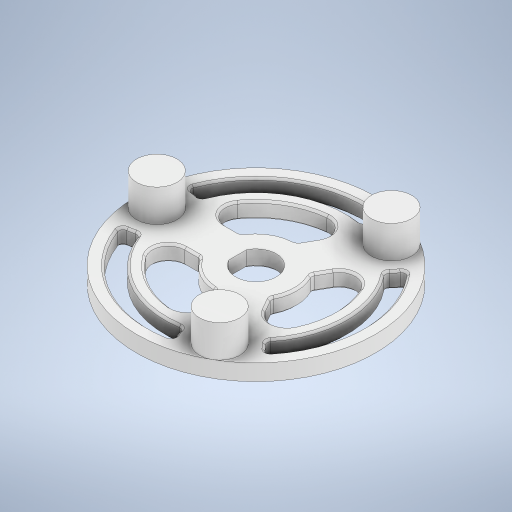
# Autodesk Inventor part: insert
Saved by Autodesk Inventor 2023 (Build 270158000, 158)
## iProperties
Created: 2022-12-06
Part Number: insert
Material: Acetal Resin, White
Document SubType Name: Modeling
Designer: Owner
Density: 1.425 g/cm^3
Appearance: Smooth - White
Mass: 2.2255 g
Surface Area: 17.3109 cm^2
Volume: 1.56175 cm^3
Author: Owner
Autodesk Inventor part; units mm, degrees
ref_plane "YZ Plane" through (0, 0, 0) normal (1, 0, 0) x (0, 1, 0)
ref_plane "XZ Plane" through (0, 0, 0) normal (0, 1, 0) x (-1, 0, 0)
ref_plane "XY Plane" through (0, 0, 0) normal (0, 0, 1) x (1, 0, 0)
sketch "Sketch1" plane through (0, 0, 0) normal (0, 1, 0) x (-1, 0, 0)
  line L0 (15.55, 0) -> (21.15, 0) construction
  line L1 (18.35, 0) -> (21.15, 0) construction
  arc A0 (2.25, 1.0897) -> (2.25, -1.0897) centre (0, 0) ccw construction
  circle A1 centre (0, 0) radius 2.25 construction
  line L2 (2.25, 0) -> (2.25, 1.0897) construction
  line L3 (2.25, 0) -> (2.25, -1.0897) construction
  line L4 (-15.5, 21.15) -> (15.5, 21.15) construction
  line L5 (21.15, 15.5) -> (21.15, -15.5) construction
  line L6 (15.5, -21.15) -> (-15.5, -21.15) construction
  line L7 (-21.15, -15.5) -> (-21.15, 15.5) construction
  line L8 (-21.15, 21.15) -> (21.15, -21.15) construction
  line L9 (21.15, 21.15) -> (-21.15, -21.15) construction
  line L10 (-15.5, 15.5) -> (15.5, 15.5) construction
  line L11 (15.5, 15.5) -> (15.5, -15.5) construction
  line L12 (15.5, -15.5) -> (-15.5, -15.5) construction
  line L13 (-15.5, -15.5) -> (-15.5, 15.5) construction
  line L14 (-15.5, 15.5) -> (15.5, -15.5) construction
  line L15 (15.5, 15.5) -> (-15.5, -15.5) construction
  circle A2 centre (15.5, 15.5) radius 1.625 construction
  circle A3 centre (15.5, -15.5) radius 1.625 construction
  circle A4 centre (-15.5, -15.5) radius 1.625 construction
  circle A5 centre (-15.5, 15.5) radius 1.625 construction
  line L16 (15.5, -15.5) -> (15.5, -21.15) construction
  line L17 (21.15, -15.5) -> (15.5, -21.15) construction
  line L18 (-15.5, -21.15) -> (-21.15, -15.5) construction
  line L19 (-21.15, 15.5) -> (-15.5, 21.15) construction
  line L20 (15.5, 21.15) -> (21.15, 15.5) construction
  line L21 (0, -15.5) -> (0, -21.15) construction
  line L22 (0, -15.5) -> (0, -18.325) construction
  line L23 (0, -18.325) -> (0, -21.15) construction
  circle A6 centre (0, 0) radius 19.7375 construction
  line L24 (-15.5, -21.15) -> (15.5, -21.15) construction
  line L25 (-13.9565, -13.9565) -> (-6.763, -21.15) construction
  line L26 (0, 0) -> (7.7782, -7.7782) construction
  line L27 (13.9565, 13.9565) -> (21.15, 6.763) construction
  line L28 (-1.1373, -19.7047) -> (0.308, -21.15) construction
  line L29 (19.7047, 1.1373) -> (21.15, -0.308) construction
  arc A7 (2.25, 1.0897) -> (2.25, -1.0897) centre (0, 0) ccw
  line L30 (2.25, 1.0897) -> (2.25, -1.0897)
  circle A8 centre (0, 0) radius 3.75
  line L31 (-19.7375, 0) -> (-17.7375, 0)
  line L32 (-19.7375, 0) -> (-14.7375, 0)
  line L33 (-17.7375, 0) -> (-6.7375, 0)
  circle A9 centre (-12.2375, 0) radius 5.5 construction
  circle A10 centre (-12.2375, 0) radius 2.5
  line L34 (-12.2375, 2.5) -> (-1.8548, 2.5) construction
  line L35 (-12.2375, -2.5) -> (-1.8548, -2.5) construction
  line L36 (3.9537, -11.848) -> (-1.2377, -2.8563) construction
  circle A11 centre (6.1187, -10.598) radius 2.5
  line L37 (8.2838, -9.348) -> (3.0924, -0.3563) construction
  circle A12 centre (6.1187, -10.598) radius 5.5 construction
  line L38 (8.2838, 9.348) -> (3.0924, 0.3563) construction
  circle A13 centre (6.1188, 10.598) radius 2.5
  line L39 (3.9537, 11.848) -> (-1.2377, 2.8563) construction
  circle A14 centre (6.1188, 10.598) radius 5.5 construction
  circle A15 centre (0, 0) radius 14.7375
  circle A16 centre (0, 0) radius 9.7375
  point P0 (-10.421, -10.421)
  point P1 (10.421, 10.421)
  point P2 (20.4274, 0.4146)
  point P3 (15.5, 12.2196)
  point P4 (15.5, 12.413)
  point P5 (-12.413, -15.5)
  point P6 (-12.2196, -15.5)
  point P7 (0, -20.842)
  point P8 (21.15, -0.308)
  point P9 (3.3687, -5.8348)
  point P10 (3.3688, 5.8348)
  dimension "d9" = 4.5
  dimension "d8" = 5
  dimension "d10" = 42.3
  dimension "d11" = 42.3
  dimension "d12" = 31
  dimension "d13" = 31
  dimension "d15" = 3.25
  dimension "d16" = 3.25
  dimension "d17" = 3.25
  dimension "d18" = 3.25
  dimension "d20" = 5
  dimension "d21" = 7.5
  dimension "d22" = 2
  dimension "d23" = 5
  dimension "d24" = 11
  dimension "d25" = 5
  dimension "d28" = 360
  dimension "d31" = 5
  constraints: 80 end point, 14 point on circle, 12 centre point, 11 coincident, 10 midpoint, 10 point on line, 7 perpendicular, 6 horizontal, 4 parallel, 4 symmetric about line, 3 collinear, 3 horizontal alignment, 2 tangent, 2 vertical, 1 concentric, 46 other
  measures "d8" diameter of A0
  measures "d10" distance of L8.end L9.end
  measures "d11" distance of L9.start L8.end
  measures "d12" distance of L11.end L12.end
  measures "d13" distance of L10.end L11.end
  measures "d15" diameter of A2
  measures "d16" diameter of A3
  measures "d17" diameter of A4
  measures "d18" diameter of A5
  measures "d20" distance from line of point (20.427, 0.415) L27
  measures "d21" diameter of A8
  measures "d22" distance of L31.start L31.end
  measures "d23" distance of L31.start L32.end
  measures "d24" distance of L31.end L33.end
  measures "d25" diameter of A10
extrude "Extrusion1" add sketch "Sketch1" along normal blind 2 contours A8 | A10 L33 | A15 A13 A16 A10 | L33 A10 | A10 A16 A11 A15 | A16 | A15 A11 A16 A13 | A13 | A11
sketch "Sketch2" plane through (0, 2, 0) normal (0, 1, 0) x (1, 0, 0)
  line L0 (15.55, 0) -> (21.15, 0) construction
  line L1 (18.35, 0) -> (21.15, 0) construction
  arc A0 (2.25, 1.0897) -> (2.25, -1.0897) centre (0, 0) ccw construction
  circle A1 centre (0, 0) radius 2.25 construction
  line L2 (2.25, 0) -> (2.25, 1.0897) construction
  line L3 (2.25, 0) -> (2.25, -1.0897) construction
  line L4 (-15.5, 21.15) -> (15.5, 21.15) construction
  line L5 (21.15, 15.5) -> (21.15, -15.5) construction
  line L6 (15.5, -21.15) -> (-15.5, -21.15) construction
  line L7 (-21.15, -15.5) -> (-21.15, 15.5) construction
  line L8 (-21.15, 21.15) -> (21.15, -21.15) construction
  line L9 (21.15, 21.15) -> (-21.15, -21.15) construction
  line L10 (-15.5, 15.5) -> (15.5, 15.5) construction
  line L11 (15.5, 15.5) -> (15.5, -15.5) construction
  line L12 (15.5, -15.5) -> (-15.5, -15.5) construction
  line L13 (-15.5, -15.5) -> (-15.5, 15.5) construction
  line L14 (-15.5, 15.5) -> (15.5, -15.5) construction
  line L15 (15.5, 15.5) -> (-15.5, -15.5) construction
  circle A2 centre (15.5, 15.5) radius 1.625 construction
  circle A3 centre (15.5, -15.5) radius 1.625 construction
  circle A4 centre (-15.5, -15.5) radius 1.625 construction
  circle A5 centre (-15.5, 15.5) radius 1.625 construction
  line L16 (15.5, -15.5) -> (15.5, -21.15) construction
  line L17 (21.15, -15.5) -> (15.5, -21.15) construction
  line L18 (-15.5, -21.15) -> (-21.15, -15.5) construction
  line L19 (-21.15, 15.5) -> (-15.5, 21.15) construction
  line L20 (15.5, 21.15) -> (21.15, 15.5) construction
  line L21 (0, -15.5) -> (0, -21.15) construction
  line L22 (0, -15.5) -> (0, -18.325) construction
  line L23 (0, -18.325) -> (0, -21.15) construction
  circle A6 centre (0, 0) radius 19.7375 construction
  line L24 (-15.5, -21.15) -> (15.5, -21.15) construction
  line L25 (-13.9565, -13.9565) -> (-6.763, -21.15) construction
  line L26 (0, 0) -> (7.7782, -7.7782) construction
  line L27 (13.9565, 13.9565) -> (21.15, 6.763) construction
  line L28 (-1.1373, -19.7047) -> (0.308, -21.15) construction
  line L29 (19.7047, 1.1373) -> (21.15, -0.308) construction
  arc A7 (2.25, 1.0897) -> (2.25, -1.0897) centre (0, 0) ccw
  line L30 (2.25, 1.0897) -> (2.25, -1.0897)
  circle A8 centre (0, 0) radius 3.75
  line L31 (-19.7375, 0) -> (-17.7375, 0)
  line L32 (-19.7375, 0) -> (-14.7375, 0)
  line L33 (-17.7375, 0) -> (-6.7375, 0)
  circle A9 centre (-12.2375, 0) radius 5.5 construction
  circle A10 centre (-12.2375, 0) radius 2.5
  line L34 (-12.2375, 2.5) -> (-1.8548, 2.5) construction
  line L35 (-12.2375, -2.5) -> (-1.8548, -2.5) construction
  line L36 (3.9537, -11.848) -> (-1.2377, -2.8563) construction
  circle A11 centre (6.1187, -10.598) radius 2.5
  line L37 (8.2838, -9.348) -> (3.0924, -0.3563) construction
  circle A12 centre (6.1187, -10.598) radius 5.5 construction
  line L38 (8.2838, 9.348) -> (3.0924, 0.3563) construction
  circle A13 centre (6.1188, 10.598) radius 2.5
  line L39 (3.9537, 11.848) -> (-1.2377, 2.8563) construction
  circle A14 centre (6.1188, 10.598) radius 5.5 construction
  circle A15 centre (0, 0) radius 14.7375
  circle A16 centre (0, 0) radius 9.7375
  point P0 (-10.421, -10.421)
  point P1 (20.4274, 0.4146)
  point P2 (10.421, 10.421)
  point P3 (15.5, 12.2196)
  point P4 (15.5, 12.413)
  point P5 (-12.413, -15.5)
  point P6 (-12.2196, -15.5)
  point P7 (0, -20.842)
  point P8 (21.15, -0.308)
  point P9 (3.3687, -5.8348)
  point P10 (3.3688, 5.8348)
  dimension "d37" = 4.5
  dimension "d36" = 5
  dimension "d38" = 42.3
  dimension "d39" = 42.3
  dimension "d40" = 31
  dimension "d41" = 31
  dimension "d42" = 3.25
  dimension "d43" = 3.25
  dimension "d44" = 3.25
  dimension "d45" = 3.25
  dimension "d46" = 5
  dimension "d47" = 7.5
  dimension "d48" = 2
  dimension "d49" = 5
  dimension "d50" = 11
  dimension "d51" = 5
  dimension "d52" = 360
  dimension "d53" = 5
  constraints: 80 end point, 14 point on circle, 12 centre point, 11 coincident, 10 midpoint, 10 point on line, 7 perpendicular, 6 horizontal, 4 parallel, 4 symmetric about line, 3 collinear, 3 horizontal alignment, 2 tangent, 2 vertical, 1 concentric, 46 other
  measures "d36" diameter of A0
  measures "d38" distance of L8.end L9.end
  measures "d39" distance of L9.start L8.end
  measures "d40" distance of L11.end L12.end
  measures "d41" distance of L10.end L11.end
  measures "d42" diameter of A2
  measures "d43" diameter of A3
  measures "d44" diameter of A4
  measures "d45" diameter of A5
  measures "d46" distance from line of point (20.427, 0.415) L27
  measures "d47" diameter of A8
  measures "d48" distance of L31.start L31.end
  measures "d49" distance of L31.start L32.end
  measures "d50" distance of L31.end L33.end
  measures "d51" diameter of A10
extrude "Extrusion2" add sketch "Sketch2" along normal blind 4 contours A10 L33 | L33 A10 | A13 | A11
sketch "Sketch4" plane through (6.1187, 2, 10.598) normal (0, 1, 0) x (1, 0, 0)
  circle A0 centre (-6.1187, 10.598) radius 14.7375 projected
  arc A1 (-14.0401, 4.9348) -> (-7.0625, 0.9063) centre (-6.1187, 10.598) ccw
  circle A2 centre (-18.3562, 10.598) radius 2.5 projected
  arc A3 (-20.8562, 10.598) -> (-15.8562, 10.598) centre (-18.3562, 10.598) ccw
  arc A4 (-1.25, 2.1651) -> (1.25, -2.1651) centre (0, 0) ccw
  arc A5 (-20.8562, 10.598) -> (1.25, -2.1651) centre (-6.1187, 10.598) ccw
  arc A6 (-3.8978, -0.8985) -> (-3.5964, -1.7509) centre (0, 0) ccw
  arc A7 (-18.507, 5.933) -> (-3.9646, -2.4631) centre (-6.1187, 10.598) ccw
  arc A8 (-16.5739, 6.4784) -> (-4.4589, -0.5162) centre (-6.1187, 10.598) ccw
  arc A9 (-18.0743, 6.6079) -> (-17.1854, 6.7732) centre (-18.3562, 10.598) ccw
  line L0 (-12.4131, 8.098) -> (-10.7285, 8.098)
  arc A10 (-8.3687, 9.5083) -> (-8.3687, 11.6877) centre (-6.1187, 10.598) ccw projected
  arc A11 (-12.4131, 8.098) -> (-14.0401, 4.9348) centre (-12.4131, 6.098) ccw
  arc A12 (-16.5739, 6.4784) -> (-17.1854, 6.7732) centre (-17.0391, 6.2951) ccw
  arc A13 (-18.0743, 6.6079) -> (-18.507, 5.933) centre (-18.0391, 6.1092) ccw
  arc A14 (-3.9646, -2.4631) -> (-3.5964, -1.7509) centre (-4.046, -1.9697) ccw
  arc A15 (-3.8978, -0.8985) -> (-4.4589, -0.5162) centre (-4.385, -1.0108) ccw
  arc A16 (-10.3095, 7.8707) -> (-10.7285, 8.098) centre (-10.7285, 7.598) ccw
  line L1 (-6.1187, 10.598) -> (-9.6187, 4.5358)
  line L2 (-6.1187, 10.598) -> (0.8813, 10.598) construction
  arc A17 (-14.0401, 4.9348) -> (-7.0625, 0.9063) centre (-6.1187, 10.598) ccw
  line L3 (-5.1366, 3.8969) -> (-5.9789, 5.3558)
  arc A18 (-7.0625, 0.9063) -> (-5.1366, 3.8969) centre (-6.8687, 2.8969) ccw
  arc A19 (-5.9789, 5.3558) -> (-6.3853, 5.6051) centre (-6.4119, 5.1058) ccw
  arc A20 (-10.3095, 7.8707) -> (-6.3853, 5.6051) centre (-6.1187, 10.598) ccw
  arc A21 (-10.3095, 7.8707) -> (-6.3853, 5.6051) centre (-6.1187, 10.598) ccw
  line L4 (-0.8065, 14.7991) -> (-1.6488, 13.3402)
  arc A22 (-1.6488, 13.3402) -> (-1.6615, 12.8636) centre (-1.2158, 13.0902) ccw
  line L5 (-6.1187, 10.598) -> (-9.6187, 16.6602) construction
  arc A23 (-1.6615, 8.3324) -> (-1.6615, 12.8636) centre (-6.1187, 10.598) ccw
  arc A24 (-1.6615, 8.3324) -> (-1.6615, 12.8636) centre (-6.1187, 10.598) ccw
  line L6 (-6.1187, 10.598) -> (0.8813, 10.598)
  arc A25 (2.7464, 6.5695) -> (2.7464, 14.6265) centre (-6.1187, 10.598) ccw
  arc A26 (2.7464, 6.5695) -> (2.7464, 14.6265) centre (-6.1187, 10.598) ccw
  arc A27 (1.25, -2.1651) -> (1.25, 23.361) centre (-6.1187, 10.598) ccw
  arc A28 (4.1154, 2.2019) -> (4.1154, 18.994) centre (-6.1187, 10.598) ccw
  arc A29 (2.6765, 3.6034) -> (2.6765, 17.5926) centre (-6.1187, 10.598) ccw
  line L7 (-0.8065, 6.3969) -> (-1.6488, 7.8558)
  arc A30 (1.25, -2.1651) -> (-1.25, 2.1651) centre (0, 0) ccw
  arc A31 (-1.6615, 8.3324) -> (-1.6488, 7.8558) centre (-1.2158, 8.1058) ccw
  arc A32 (3.3145, 2.2392) -> (2.727, 2.9264) centre (0, 0) ccw
  arc A33 (-0.8065, 6.3969) -> (2.7464, 6.5695) centre (0.9255, 7.3969) ccw
  arc A34 (2.6765, 3.6034) -> (2.727, 2.9264) centre (3.0679, 3.2922) ccw
  arc A35 (3.3145, 2.2392) -> (4.1154, 2.2019) centre (3.7288, 2.5191) ccw
  arc A36 (2.727, 18.2696) -> (3.3145, 18.9568) centre (0, 21.196) ccw
  arc A37 (2.727, 18.2696) -> (2.6765, 17.5926) centre (3.0679, 17.9038) ccw
  arc A38 (4.1154, 18.994) -> (3.3145, 18.9568) centre (3.7288, 18.6769) ccw
  arc A39 (-1.25, 19.0309) -> (1.25, 23.361) centre (0, 21.196) ccw
  arc A40 (2.7464, 14.6265) -> (-0.8065, 14.7991) centre (0.9255, 13.7991) ccw
  line L8 (-12.4131, 13.098) -> (-10.7285, 13.098)
  arc A41 (-10.7285, 13.098) -> (-10.3095, 13.3253) centre (-10.7285, 13.598) ccw
  line L9 (-6.1187, 10.598) -> (-9.6187, 4.5358) construction
  arc A42 (-6.3853, 15.5909) -> (-10.3095, 13.3253) centre (-6.1187, 10.598) ccw
  arc A43 (-6.3853, 15.5909) -> (-10.3095, 13.3253) centre (-6.1187, 10.598) ccw
  line L10 (-6.1187, 10.598) -> (-9.6187, 16.6602)
  arc A44 (-7.0625, 20.2896) -> (-14.0401, 16.2612) centre (-6.1187, 10.598) ccw
  arc A45 (-7.0625, 20.2896) -> (-14.0401, 16.2612) centre (-6.1187, 10.598) ccw
  arc A46 (1.25, 23.361) -> (-20.8562, 10.598) centre (-6.1187, 10.598) ccw
  arc A47 (-3.9646, 23.659) -> (-18.507, 15.263) centre (-6.1187, 10.598) ccw
  arc A48 (-4.4589, 21.7122) -> (-16.5739, 14.7176) centre (-6.1187, 10.598) ccw
  line L11 (-5.1366, 17.2991) -> (-5.9789, 15.8402)
  arc A49 (1.25, 23.361) -> (-1.25, 19.0309) centre (0, 21.196) ccw
  arc A50 (-6.3853, 15.5909) -> (-5.9789, 15.8402) centre (-6.4119, 16.0902) ccw
  arc A51 (-3.5964, 22.9468) -> (-3.8978, 22.0944) centre (0, 21.196) ccw
  arc A52 (-5.1366, 17.2991) -> (-7.0625, 20.2896) centre (-6.8687, 18.2991) ccw
  arc A53 (-4.4589, 21.7122) -> (-3.8978, 22.0944) centre (-4.385, 22.2067) ccw
  arc A54 (-3.5964, 22.9468) -> (-3.9646, 23.659) centre (-4.046, 23.1657) ccw
  arc A55 (-17.1854, 14.4228) -> (-18.0743, 14.588) centre (-18.3562, 10.598) ccw
  arc A56 (-17.1854, 14.4228) -> (-16.5739, 14.7176) centre (-17.0391, 14.9009) ccw
  arc A57 (-18.507, 15.263) -> (-18.0743, 14.588) centre (-18.0391, 15.0868) ccw
  arc A58 (-15.8562, 10.598) -> (-20.8562, 10.598) centre (-18.3562, 10.598) ccw
  arc A59 (-14.0401, 16.2612) -> (-12.4131, 13.098) centre (-12.4131, 15.098) ccw
  point P0 (-10.4489, 8.098)
  point P1 (-1.7886, 8.098)
  point P2 (-6.1187, 15.598)
  dimension "d60" = 2
  dimension "d62" = 0.5
  dimension "d63" = 4
  dimension "d64" = 13.2375
  dimension "d65" = 11.2375
  dimension "d67" = 0.5
  dimension "d68" = 7
  dimension "d69" = 120
  dimension "d70" = 5
  dimension "d71" = 8.4329
  dimension "d72" = 2.5
  dimension "d75" = 360
  constraints: 119 point on circle, 57 centre point, 24 end point, 17 tangent, 6 symmetric about line, 5 equal radius, 4 coincident, 3 point on line, 1 equal length, 1 horizontal, 1 horizontal alignment, 182 other
  measures "d60" radius of A11
  measures "d62" radius of A12
  measures "d63" radius of A6
  measures "d64" radius of A7
  measures "d65" radius of A8
  measures "d67" radius of A16
  measures "d68" distance of L1.start L1.end
  measures "d69" angle of L1 L2
  measures "d70" radius of A21
  measures "d71" distance from line of A4.start L2
  measures "d72" distance from line of point (-10.449, 8.098) L3
extrude "Extrusion3" cut sketch "Sketch4" against normal blind 3.75 contours A11 L0 A16 A20 A19 L3 A18 A1 | A6 A14 A7 A13 A9 A12 A8 A15 | A40 A25 A33 L7 A31 A23 A22 L4 | A35 A32 A34 A29 A37 A36 A38 A28 | A59 A44 A52 L11 A50 A42 A41 L8 | A54 A51 A53 A48 A56 A55 A57 A47
chamfer "Chamfer1" distance 0.25 angle 45 98 edges at (-6.6187, 2, -11.464) (2.5169, 2, -12.7973) (2.3475, 2, -11.9312) (2.0152, 2, -11.1955) (-5.6187, 2, -9.732) (-10.7032, 2, -3.8525) (-11.5065, 2, -3.9326) (-12.3413, 2, -4.219) (-4.8687, 2, -8.4329) (0.9316, 2, -8.7839) (0.561, 2, -5.9716) (-0.0317, 2, -5.066) (-2.5, 2, -4.3301) (-4.3714, 2, -2.5605) (-5.4521, 2, -2.5) (-8.0729, 2, -3.5852) (-8.0729, 2, 3.5852) (-5.4521, 2, 2.5) (-4.3714, 2, 2.5605) (-2.5, 2, 4.3301) (-0.0317, 2, 5.066) (0.561, 2, 5.9716) (0.9316, 2, 8.7839) (-4.8687, 2, 8.4329) (-11.5065, 2, 3.9326) (-10.7032, 2, 3.8525) (-5.6188, 2, 9.732) (2.0152, 2, 11.1955) (2.3475, 2, 11.9312) (2.5169, 2, 12.7973) (-6.6188, 2, 11.464) (-12.3413, 2, 4.219) (-11.5065, 0, 3.9326) (-12.3413, 0, 4.219) (-6.6188, 0, 11.464) (2.5169, 0, 12.7973) (2.3475, 0, 11.9312) (2.0152, 0, 11.1955) (-5.6187, 0, 9.732) (-10.7032, 0, 3.8525) (-8.0729, 0, 3.5852) (-4.8687, 0, 8.4329) (0.9316, 0, 8.7839) (0.561, 0, 5.9716) (-0.0317, 0, 5.066) (-2.5, 0, 4.3301) (-4.3714, 0, 2.5605) (-5.4521, 0, 2.5) (-4.8687, 0, -8.4329) (-8.0729, 0, -3.5852) (-5.4521, 0, -2.5) (-4.3714, 0, -2.5605) (-2.5, 0, -4.3301) (-0.0317, 0, -5.066) (0.561, 0, -5.9716) (0.9316, 0, -8.7839) (4.8911, 0, -3.4716) (4.4031, 0, -2.5055) (5, 0, 0) (4.4031, 0, 2.5055) (4.8911, 0, 3.4716) (7.1413, 0, 5.1987) (9.7375, 0, 0) (7.1413, 0, -5.1987) (4.8911, 2, -3.4716) (7.1413, 2, -5.1987) (9.7375, 2, 0) (7.1413, 2, 5.1987) (4.8911, 2, 3.4716) (4.4031, 2, 2.5055) (5, 2, 0) (4.4031, 2, -2.5055) (11.2375, 2, 0) (8.688, 2, -7.343) (9.159, 2, -7.9986) (9.8244, 2, -8.5784) (13.2375, 2, 0) (9.8244, 2, 8.5784) (9.159, 2, 7.9986) (8.688, 2, 7.343) (9.159, 0, -7.9986) (8.688, 0, -7.343) (11.2375, 0, 0) (8.688, 0, 7.343) (9.159, 0, 7.9986) (9.8244, 0, 8.5784) (13.2375, 0, 0) (9.8244, 0, -8.5784) (-6.6187, 0, -11.464) (-12.3413, 0, -4.219) (-11.5065, 0, -3.9326) (-10.7032, 0, -3.8525) (-5.6187, 0, -9.732) (2.0152, 0, -11.1955) (2.3475, 0, -11.9312) (2.5169, 0, -12.7973) (2.5, 0, 0) (-2.25, 0, 0)
body "Solid1"
